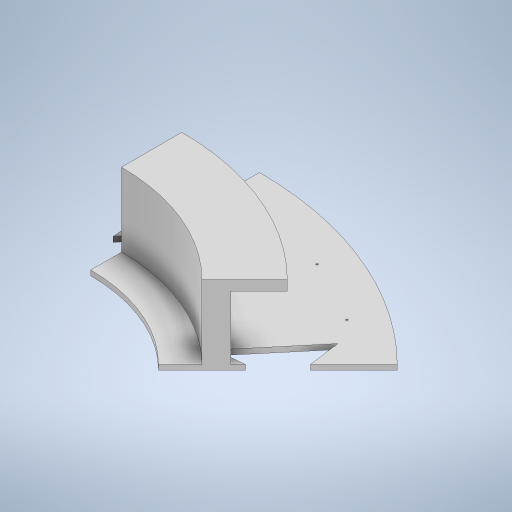
# Autodesk Inventor part: Carousel Base Plate v2
Saved by Autodesk Inventor 2023 (Build 270158000, 158)
## iProperties
Created: 2023-02-03
Part Number: Carousel Base Plate v2
Material: Generic
Document SubType Name: Modeling
Designer: cheng
Density: 1 g/cm^3
Appearance: Default
Author: cheng
Autodesk Inventor part; units mm, degrees
ref_plane "YZ Plane" through (0, 0, 0) normal (1, 0, 0) x (0, 1, 0)
ref_plane "XZ Plane" through (0, 0, 0) normal (0, 1, 0) x (-1, 0, 0)
ref_plane "XY Plane" through (0, 0, 0) normal (0, 0, 1) x (1, 0, 0)
sketch "Sketch1" plane through (0, 0, 0) normal (0, 1, 0) x (-1, 0, 0)
  circle A0 centre (0, 0) radius 160
  circle A1 centre (0, 0) radius 325
  line L0 (0, 0) -> (0, -325)
  line L1 (0, 0) -> (-229.8097, -229.8097)
  line L2 (0, 0) -> (28.3256, -323.7633)
  line L3 (0, 0) -> (-208.906, -248.9644)
  circle A2 centre (0, 0) radius 285
  circle A3 centre (0, 0) radius 265
  circle A4 centre (0, 0) radius 200
  circle A5 centre (0, 0) radius 220
  line L4 (0, -220) -> (17.4311, -199.2389)
  line L5 (0, -265) -> (24.8394, -283.9155)
  line L6 (-128.5575, -153.2089) -> (-155.5635, -155.5635)
  line L7 (-187.3833, -187.3833) -> (-183.1945, -218.3227)
  point P0 (-113.1371, -113.1371)
  point P1 (0, -160)
  dimension "d0" = 650
  dimension "d1" = 320
  dimension "d2" = 45
  dimension "d13" = 40
  dimension "d14" = 40
  dimension "d15" = 20
  dimension "d16" = 20
  dimension "d17" = 5
  dimension "d18" = 5
  constraints: 16 end point, 12 point on circle, 8 point on line, 6 centre point, 6 coincident, 1 vertical
  measures "d0" diameter of A1
  measures "d1" diameter of A0
  measures "d2" angle of L1 L0
  measures "d13" radial gap between concentric circles of A0 A4
  measures "d14" radial gap between concentric circles of A1 A2
  measures "d15" radial gap between concentric circles of A5 A4
  measures "d16" radial gap between concentric circles of A2 A3
  measures "d17" angle of L0 L2
  measures "d18" angle of L1 L3
extrude "Extrusion1" add sketch "Sketch1" along normal blind 5 contours A0 L3 A4 L1 | A0 L0 A4 L3 | A4 L6 L1 | L2 A5 L4 | A4 L0 A5 L3 | L2 A3 L0 A5 | L0 A3 L3 A5 | L7 A2 L1 | L2 L5 A3 | L0 A2 L3 A3 | A2 L3 A1 L1 | A2 L0 A1 L3
sketch "Sketch2" plane through (0, 5, 0) normal (0, 1, 0) x (1, 0, 0)
  arc A0 (229.8097, 229.8097) -> (0, 325) centre (0, 0) ccw projected
  line L0 (0, 325) -> (0, 265) projected
  arc A1 (113.1371, 113.1371) -> (0, 160) centre (0, 0) ccw projected
  line L1 (113.1371, 113.1371) -> (155.5635, 155.5635) projected
  circle A2 centre (0, 0) radius 190
  circle A3 centre (0, 0) radius 210
  line L2 (155.5635, 155.5635) -> (128.5575, 153.2089) projected
  line L3 (128.5575, 153.2089) -> (183.1945, 218.3227) projected
  line L4 (183.1945, 218.3227) -> (187.3833, 187.3833) projected
  line L5 (187.3833, 187.3833) -> (229.8097, 229.8097) projected
  line L6 (0, 265) -> (-24.8394, 283.9155) projected
  line L7 (-24.8394, 283.9155) -> (-17.4311, 199.2389) projected
  line L8 (-17.4311, 199.2389) -> (0, 220) projected
  line L9 (0, 220) -> (0, 160) projected
  point P0 (148.4924, 148.4924)
  point P1 (0, 210)
  point P2 (0, 190)
  point P3 (134.3503, 134.3503)
  point P4 (0, 190)
  point P5 (0, 210)
  point P6 (-8.542, 209.8262)
  point P7 (-18.3027, 209.2009)
  point P8 (142.3294, 154.4096)
  point P9 (134.9854, 160.8693)
  dimension "d5" = 420
  dimension "d6" = 20
  constraints: 2 centre point, 2 coincident
  measures "d5" diameter of A3
  measures "d6" radial gap between concentric circles of A3 A2
extrude "Extrusion2" add sketch "Sketch2" along normal blind 62 contours L3 L2 A3 L1 A2 L9 | A3 L2 L3
sketch "Sketch3" plane through (0, 67, 0) normal (0, 1, 0) x (1, 0, 0)
  line L0 (134.3503, 134.3503) -> (148.4924, 148.4924) projected
  arc A0 (148.4924, 148.4924) -> (0, 210) centre (0, 0) ccw projected
  circle A1 centre (0, 0) radius 190
  circle A2 centre (0, 0) radius 249
  line L1 (0, 190) -> (0, 160) projected
  line L2 (113.1371, 113.1371) -> (134.3503, 134.3503) projected
  arc A3 (148.4924, 148.4924) -> (142.3294, 154.4096) centre (0, 0) ccw projected
  line L3 (148.4924, 148.4924) -> (155.5635, 155.5635) projected
  arc A4 (229.8097, 229.8097) -> (0, 325) centre (0, 0) ccw projected
  line L4 (0, 220) -> (0, 210) projected
  line L5 (-17.4311, 199.2389) -> (0, 220) projected
  line L6 (0, 325) -> (0, 265) projected
  arc A5 (134.9854, 160.8693) -> (0, 210) centre (0, 0) ccw projected
  line L7 (134.9854, 160.8693) -> (183.1945, 218.3227) projected
  line L8 (183.1945, 218.3227) -> (187.3833, 187.3833) projected
  line L9 (0, 265) -> (-24.8394, 283.9155) projected
  line L10 (-24.8394, 283.9155) -> (-17.4311, 199.2389) projected
  arc A6 (148.4924, 148.4924) -> (142.3294, 154.4096) centre (0, 0) ccw projected
  line L11 (-17.4311, 199.2389) -> (0, 220) projected
  arc A7 (134.9854, 160.8693) -> (0, 210) centre (0, 0) ccw projected
  line L12 (134.9854, 160.8693) -> (183.1945, 218.3227) projected
  line L13 (183.1945, 218.3227) -> (187.3833, 187.3833) projected
  arc A8 (229.8097, 229.8097) -> (0, 325) centre (0, 0) ccw projected
  line L14 (0, 325) -> (0, 265) projected
  line L15 (0, 265) -> (-24.8394, 283.9155) projected
  line L16 (-24.8394, 283.9155) -> (-17.4311, 199.2389) projected
  line L17 (187.3833, 187.3833) -> (229.8097, 229.8097) projected
  arc A9 (134.3503, 134.3503) -> (0, 190) centre (0, 0) ccw projected
  line L18 (0, 190) -> (0, 160) projected
  arc A10 (113.1371, 113.1371) -> (0, 160) centre (0, 0) ccw projected
  line L19 (113.1371, 113.1371) -> (134.3503, 134.3503) projected
  line L20 (155.5635, 155.5635) -> (142.3294, 154.4096) projected
  line L21 (187.3833, 187.3833) -> (229.8097, 229.8097) projected
  line L22 (0, 220) -> (0, 210) projected
  arc A11 (134.3503, 134.3503) -> (0, 190) centre (0, 0) ccw projected
  arc A12 (113.1371, 113.1371) -> (0, 160) centre (0, 0) ccw projected
  line L23 (148.4924, 148.4924) -> (155.5635, 155.5635) projected
  line L24 (155.5635, 155.5635) -> (142.3294, 154.4096) projected
  arc A13 (134.3503, 134.3503) -> (0, 190) centre (0, 0) ccw projected
  line L25 (0, 210) -> (0, 190) projected
  line L26 (0, 0) -> (229.8097, 229.8097)
  arc A14 (229.8097, 229.8097) -> (0, 325) centre (0, 0) ccw projected
  line L27 (0, 0) -> (0, 325)
  point P0 (176.0696, 176.0696)
  point P1 (0, 249)
  point P2 (-18.3027, 209.2009)
  point P3 (-21.7018, 248.0525)
  point P4 (160.0541, 190.7451)
  point P5 (0, 210)
  point P6 (-8.542, 209.8262)
  point P7 (0, 210)
  point P8 (0, 210)
  point P9 (176.0696, 176.0696)
  point P10 (0, 249)
  dimension "d12" = 59
  constraints: 4 end point, 2 centre point, 2 coincident, 1 collinear
  measures "d12" radial gap between concentric circles of A2 A1
extrude "Extrusion3" add sketch "Sketch3" along normal blind 10 contours A1 L25 A0 L0 | A0 L20 L3 | A0 L7 A2 L26 L20 | L4 L27 A2 L7 A0
sketch "Sketch5" plane through (0, 5, 0) normal (0, 1, 0) x (1, 0, 0)
  circle A0 centre (0, 0) radius 295
  arc A1 (134.9854, 160.8693) -> (0, 210) centre (0, 0) ccw projected
  line L0 (134.9854, 160.8693) -> (183.1945, 218.3227) projected
  line L1 (183.1945, 218.3227) -> (187.3833, 187.3833) projected
  line L2 (187.3833, 187.3833) -> (229.8097, 229.8097) projected
  arc A2 (229.8097, 229.8097) -> (0, 325) centre (0, 0) ccw projected
  line L3 (0, 325) -> (0, 265) projected
  line L4 (0, 265) -> (-24.8394, 283.9155) projected
  line L5 (-24.8394, 283.9155) -> (-17.4311, 199.2389) projected
  line L6 (-17.4311, 199.2389) -> (0, 220) projected
  line L7 (0, 220) -> (0, 210) projected
  point P0 (40.9671, 292.1416)
  point P1 (167.4373, 242.878)
  point P2 (105.8364, 275.361)
  dimension "d26" = 30
  constraints: 3 point on circle, 1 centre point, 1 coincident
  measures "d26" radial gap between concentric circles of A0 A2
hole "Hole1" at (40.9671, 5, -292.1416) at (167.4373, 5, -242.878) at (105.8364, 5, -275.361) direction (0, -1, 0) diameter 1.7551 end through all thread size "2-64 UNF" class "2B" standard "ANSI Unified Screw Threads"
body "Solid1"
